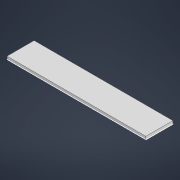
# Autodesk Inventor part: bottom
Saved by Autodesk Inventor 2022 (Build 260153000, 153)
## iProperties
Created: 2022-04-08
Part Number: bottom
Material: Типовые
Document SubType Name: Modeling
Designer: Kalugin_a
Density: 1 g/cm^3
Appearance: По умолчанию
Author: Kalugin_a
Autodesk Inventor part; units mm, degrees
ref_plane "YZ Plane" through (0, 0, 0) normal (1, 0, 0) x (0, 1, 0)
ref_plane "XZ Plane" through (0, 0, 0) normal (0, 1, 0) x (-1, 0, 0)
ref_plane "XY Plane" through (0, 0, 0) normal (0, 0, 1) x (1, 0, 0)
sketch "Эскиз1" plane through (0, 0, 0) normal (0, 1, 0) x (-1, 0, 0)
  line L0 (0, 0) -> (600, 0)
  line L1 (600, 0) -> (600, -117)
  line L2 (600, -117) -> (0, -117)
  line L3 (0, -117) -> (0, 0)
  constraints: 8 end point, 2 parallel, 1 horizontal, 1 perpendicular
extrude "Выдавливание1" add sketch "Эскиз1" along normal blind 12
